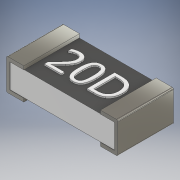
# Autodesk Inventor part: 21-1001
Saved by Autodesk Inventor 2018 (Build 220112000, 112)
## iProperties
Created: 2019-09-21
Part Number: 21-1001
Material: Copper
Document SubType Name: Modeling
Designer: Bradley
Density: 8.94 g/cm^3
Appearance: Smooth - White
Author: Bradley
Autodesk Inventor part; units mm, degrees
ref_plane "YZ Plane" through (0, 0, 0) normal (1, 0, 0) x (0, 1, 0)
ref_plane "XZ Plane" through (0, 0, 0) normal (0, 1, 0) x (-1, 0, 0)
ref_plane "XY Plane" through (0, 0, 0) normal (0, 0, 1) x (1, 0, 0)
sketch "Sketch1" plane through (0, 0, 0) normal (0, 1, 0) x (-1, 0, 0)
  line L0 (0.75, 0.175) -> (-0.75, 0.175)
  line L1 (-0.75, 0.175) -> (-0.75, -0.175)
  line L2 (-0.75, -0.175) -> (0.75, -0.175)
  line L3 (0.75, -0.175) -> (0.75, 0.175)
  line L4 (0.55, 0.175) -> (0.55, 0.225)
  line L5 (0.55, 0.225) -> (0.8, 0.225)
  line L6 (0.8, 0.225) -> (0.8, -0.225)
  line L7 (0.8, -0.225) -> (0.55, -0.225)
  line L8 (0.55, -0.225) -> (0.55, -0.175)
  line L9 (-0.55, 0.175) -> (-0.55, 0.225)
  line L10 (-0.55, 0.225) -> (-0.8, 0.225)
  line L11 (-0.8, 0.225) -> (-0.8, -0.225)
  line L12 (-0.8, -0.225) -> (-0.55, -0.225)
  line L13 (-0.55, -0.175) -> (-0.55, -0.225)
  line L14 (0.55, 0.175) -> (-0.55, 0.175)
  point P0 (0, 0)
  point P1 (0, 0.175)
  point P2 (0.75, 0)
  dimension "d0" = 1.6
  dimension "d1" = 0.05
  dimension "d2" = 0.05
  dimension "d3" = 0.45
  dimension "d4" = 0.25
  constraints: 30 end point, 12 point on line, 7 perpendicular, 3 collinear, 3 midpoint, 2 parallel, 1 horizontal, 1 horizontal alignment, 1 vertical, 1 vertical alignment
  measures "d0" distance between parallel lines of L11 L6
  measures "d1" distance of L7.end L8.end
  measures "d2" distance between parallel lines of L6 L3
  measures "d3" distance of L5.end L6.end
  measures "d4" distance of L6.end L7.end
extrude "Extrusion1" add sketch "Sketch1" along normal mid plane 0.8 contours L0 L4 L5 L6 L7 L8 L2 L3 | L0 L1 L2 L13 L12 L11 L10 L9
extrude "Extrusion2" add sketch "Sketch1" along normal mid plane 0.79 contours L3 L2 L1 L0
sketch "Sketch2" plane through (-0.55, -0.395, 0.175) normal (0, 0, 1) x (1, 0, 0)
  line L0 (0, 0) -> (0, 0.79) projected
  line L1 (1.1, 0) -> (0, 0) projected
  line L2 (1.1, 0) -> (1.1, 0.79) projected
  line L3 (0, 0.79) -> (1.1, 0.79) projected
  line L4 (0, 0.395) -> (1.1, 0.395) construction
  line L5 (0.3391, 0.195) -> (0.0925, 0.195)
  line L6 (0.0925, 0.195) -> (0.0925, 0.2517)
  spline S0 degree 2 poles (0.0925, 0.2517) (0.119, 0.2767) (0.1664, 0.323) (0.1891, 0.348) knots 0 0 0 1 2 2 2
  spline S1 degree 2 poles (0.1891, 0.348) (0.2348, 0.3982) (0.2682, 0.4585) (0.2682, 0.4906) knots 0 0 0 1 2 2 2
  spline S2 degree 2 poles (0.2682, 0.4906) (0.2682, 0.5075) (0.2578, 0.5328) (0.2484, 0.5409) knots 0 0 0 1 2 2 2
  spline S3 degree 2 poles (0.2484, 0.5409) (0.239, 0.549) (0.2143, 0.5571) (0.1994, 0.5571) knots 0 0 0 1 2 2 2
  spline S4 degree 2 poles (0.1994, 0.5571) (0.1852, 0.5571) (0.156, 0.5499) (0.1427, 0.5444) knots 0 0 0 1 2 2 2
  spline S5 degree 2 poles (0.1427, 0.5444) (0.1314, 0.5399) (0.1103, 0.5269) (0.1038, 0.5224) knots 0 0 0 1 2 2 2
  line L7 (0.1038, 0.5224) -> (0.1009, 0.5224)
  line L8 (0.1009, 0.5224) -> (0.1009, 0.5794)
  spline S6 degree 2 poles (0.1009, 0.5794) (0.1174, 0.5875) (0.1767, 0.6034) (0.2033, 0.6034) knots 0 0 0 1 2 2 2
  spline S7 degree 2 poles (0.2033, 0.6034) (0.2594, 0.6034) (0.3226, 0.5441) (0.3226, 0.4935) knots 0 0 0 1 2 2 2
  spline S8 degree 2 poles (0.3226, 0.4935) (0.3226, 0.4699) (0.3116, 0.4303) (0.3019, 0.4135) knots 0 0 0 1 2 2 2
  spline S9 degree 2 poles (0.3019, 0.4135) (0.2921, 0.396) (0.2639, 0.3616) (0.2484, 0.3451) knots 0 0 0 1 2 2 2
  spline S10 degree 2 poles (0.2484, 0.3451) (0.2231, 0.3175) (0.1612, 0.2585) (0.1427, 0.2414) knots 0 0 0 1 2 2 2
  line L9 (0.1427, 0.2414) -> (0.3391, 0.2414)
  line L10 (0.3391, 0.2414) -> (0.3391, 0.195)
  spline S11 degree 2 poles (0.6416, 0.395) (0.6416, 0.2874) (0.579, 0.1866) (0.5139, 0.1866) knots 0 0 0 1 2 2 2
  spline S12 degree 2 poles (0.5139, 0.1866) (0.4477, 0.1866) (0.3858, 0.2893) (0.3858, 0.3947) knots 0 0 0 1 2 2 2
  spline S13 degree 2 poles (0.3858, 0.3947) (0.3858, 0.5029) (0.4484, 0.6031) (0.5139, 0.6031) knots 0 0 0 1 2 2 2
  spline S14 degree 2 poles (0.5139, 0.6031) (0.5797, 0.6031) (0.6416, 0.4994) (0.6416, 0.395) knots 0 0 0 1 2 2 2
  spline S15 degree 2 poles (0.5729, 0.2731) (0.5806, 0.2929) (0.5871, 0.3538) (0.5871, 0.395) knots 0 0 0 1 2 2 2
  spline S16 degree 2 poles (0.5871, 0.395) (0.5871, 0.4362) (0.5806, 0.4968) (0.5725, 0.5172) knots 0 0 0 1 2 2 2
  spline S17 degree 2 poles (0.5725, 0.5172) (0.5644, 0.5376) (0.5362, 0.5587) (0.5139, 0.5587) knots 0 0 0 1 2 2 2
  spline S18 degree 2 poles (0.5139, 0.5587) (0.4915, 0.5587) (0.4626, 0.5376) (0.4542, 0.5166) knots 0 0 0 1 2 2 2
  spline S19 degree 2 poles (0.4542, 0.5166) (0.4461, 0.4961) (0.4403, 0.4339) (0.4403, 0.3947) knots 0 0 0 1 2 2 2
  spline S20 degree 2 poles (0.4403, 0.3947) (0.4403, 0.3525) (0.4455, 0.2961) (0.4539, 0.2741) knots 0 0 0 1 2 2 2
  spline S21 degree 2 poles (0.4539, 0.2741) (0.4617, 0.2533) (0.4905, 0.231) (0.5139, 0.231) knots 0 0 0 1 2 2 2
  spline S22 degree 2 poles (0.5139, 0.231) (0.5359, 0.231) (0.5647, 0.2521) (0.5729, 0.2731) knots 0 0 0 1 2 2 2
  spline S23 degree 2 poles (1.0195, 0.3947) (1.0195, 0.3399) (0.9751, 0.2517) (0.9378, 0.2271) knots 0 0 0 1 2 2 2
  spline S24 degree 2 poles (0.9378, 0.2271) (0.9074, 0.208) (0.8448, 0.195) (0.7962, 0.195) knots 0 0 0 1 2 2 2
  line L11 (0.7962, 0.195) -> (0.7041, 0.195)
  line L12 (0.7041, 0.195) -> (0.7041, 0.595)
  line L13 (0.7041, 0.595) -> (0.7952, 0.595)
  spline S25 degree 2 poles (0.7952, 0.595) (0.8516, 0.595) (0.9158, 0.5781) (0.9385, 0.5632) knots 0 0 0 1 2 2 2
  spline S26 degree 2 poles (0.9385, 0.5632) (0.9771, 0.5376) (1.0195, 0.453) (1.0195, 0.3947) knots 0 0 0 1 2 2 2
  spline S27 degree 2 poles (0.9641, 0.3953) (0.9641, 0.4414) (0.9336, 0.5065) (0.9035, 0.525) knots 0 0 0 1 2 2 2
  spline S28 degree 2 poles (0.9035, 0.525) (0.8821, 0.5376) (0.8338, 0.549) (0.7978, 0.549) knots 0 0 0 1 2 2 2
  line L14 (0.7978, 0.549) -> (0.7573, 0.549)
  line L15 (0.7573, 0.549) -> (0.7573, 0.241)
  line L16 (0.7573, 0.241) -> (0.7978, 0.241)
  spline S29 degree 2 poles (0.7978, 0.241) (0.8331, 0.241) (0.8866, 0.2524) (0.9083, 0.2676) knots 0 0 0 1 2 2 2
  spline S30 degree 2 poles (0.9083, 0.2676) (0.9362, 0.2864) (0.9641, 0.3486) (0.9641, 0.3953) knots 0 0 0 1 2 2 2
  point P0 (0.55, 0.395)
  constraints: 2 end point, 2 midpoint, 1 horizontal
extrude "Extrusion3" add sketch "Sketch2" along normal blind 0.02 contours L5 L6 S0 S1 S2 S3 S4 S5 L7 L8 S6 S7 S8 S9 S10 L9 L10 | S11 S12 S13 S14 | S23 S24 L11 L12 L13 S25 S26
fillet "Fillet1" radius 0.02 4 edges at (-0.8, 0, 0.225) (-0.8, 0, -0.225) (0.8, 0, 0.225) (0.8, 0, -0.225)
equation "\"d2\" = d1"
body "Solid1"
